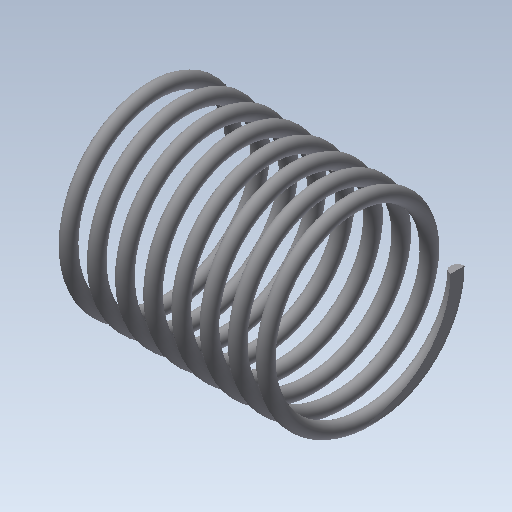
# Autodesk Inventor part: Compression Spring 16
Saved by Autodesk Inventor 2020 (Build 240168000, 168)
## iProperties
Created: 2015-04-18
Part Number: Compression Spring 16
Material: Generic
Document SubType Name: Modeling
Designer: Station9
Density: 1 g/cm^3
Appearance: Default
Mass: 0.479238 g
Surface Area: 15.5011 cm^2
Volume: 0.479238 cm^3
Author: Station9
Autodesk Inventor part; units mm, degrees
ref_plane "YZ Plane" through (0, 0, 0) normal (1, 0, 0) x (0, 1, 0)
ref_plane "XZ Plane" through (0, 0, 0) normal (0, 1, 0) x (-1, 0, 0)
ref_plane "XY Plane" through (0, 0, 0) normal (0, 0, 1) x (1, 0, 0)
sketch "Sketch1" plane through (0, 0, 0) normal (0, 1, 0) x (-1, 0, 0)
  circle A0 centre (0, -7.875) radius 0.625
  line L0 (0, 0) -> (-20, 0)
  dimension "d0" = 1.25
  dimension "d1" = 7.875
  dimension "d2" = 0
  dimension "d3" = 20
  constraints: 2 end point, 1 centre point, 1 horizontal
  measures "d0" diameter of A0
  measures "d1" distance of A0.centre L0.start
  measures "d2" horizontal distance of L0.start A0.centre
  measures "d3" distance of L0.start L0.end
coil "Coil1" sketch "Sketch1" operation add axis through (0, 0, 0) along (1, 0, 0) pitch 2.5 turns 8 hand right
sketch "Sketch2" plane through (0, 0, 0) normal (0, 0, 1) x (1, 0, 0)
  line L0 (28.4123, -11.9499) -> (20, -11.9499)
  line L1 (20, -11.9499) -> (20, 18.9136)
  line L2 (20, 18.9136) -> (28.4123, 18.9136)
  line L3 (28.4123, 18.9136) -> (28.4123, -11.9499)
  line L4 (0, 19.5265) -> (-5.961, 19.5265)
  line L5 (-5.961, 19.5265) -> (-5.961, -16.0167)
  line L6 (-5.961, -16.0167) -> (0, -16.0167)
  line L7 (0, -16.0167) -> (0, 19.5265)
  line L8 (20.625, 0) -> (19.375, 0) projected
  line L9 (-0.625, 0) -> (0.625, 0) projected
  line L10 (0, 0) -> (20, 0)
  line L11 (10, 0) -> (10, 15.9465)
  point P0 (18.75, -7.875)
  point P1 (17.5, 7.875)
  point P2 (16.25, -7.875)
  point P3 (15, 7.875)
  point P4 (13.75, -7.875)
  point P5 (12.5, 7.875)
  point P6 (11.25, -7.875)
  point P7 (10, 7.875)
  point P8 (8.75, -7.875)
  point P9 (7.5, 7.875)
  point P10 (8.875, -7.875)
  point P11 (7.875, 7.875)
  point P12 (6.875, -7.875)
  point P13 (5.875, 7.875)
  point P14 (4.875, -7.875)
  point P15 (3.875, 7.875)
  point P16 (2.875, -7.875)
  point P17 (1.875, 7.875)
  point P18 (0.875, -7.875)
  point P19 (-0.125, 7.875)
  point P20 (6.25, -7.875)
  point P21 (5, 7.875)
  point P22 (3.75, -7.875)
  point P23 (2.5, 7.875)
  point P24 (1.25, -7.875)
  point P25 (0, 7.875)
  dimension "d12" = 20
  dimension "d13" = 10
  constraints: 20 end point, 4 parallel, 2 horizontal, 2 midpoint, 2 perpendicular, 1 vertical, 16 other
  measures "d12" distance between parallel lines of L1 L7
  measures "d13" distance between parallel lines of L11 L1
extrude "Extrusion1" cut sketch "Sketch2" along normal mid plane 51.25
body "Solid1"
